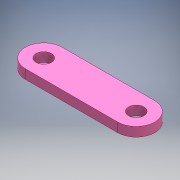
# Autodesk Inventor part: 240614_체인1
Saved by Autodesk Inventor 2016 (Build 200138000, 138)
## iProperties
Created: 2024-06-14
Part Number: 240614_체인1
Material: 일반
Document SubType Name: Modeling
Designer: pc
Density: 1 g/cm^3
Appearance: 분홍색
Author: pc
Autodesk Inventor part; units mm, degrees
ref_plane "YZ Plane" through (0, 0, 0) normal (1, 0, 0) x (0, 1, 0)
ref_plane "XZ Plane" through (0, 0, 0) normal (0, 1, 0) x (-1, 0, 0)
ref_plane "XY Plane" through (0, 0, 0) normal (0, 0, 1) x (1, 0, 0)
sketch "스케치1" plane through (0, 0, 0) normal (0, 0, 1) x (1, 0, 0)
  line L0 (-15, 0) -> (15, 0) construction
  line L1 (-15, -6) -> (15, -6)
  line L2 (15, 6) -> (-15, 6)
  arc A0 (-15, 6) -> (-15, -6) centre (-15, 0) ccw
  arc A1 (15, -6) -> (15, 6) centre (15, 0) ccw
  circle A2 centre (15, 0) radius 2.5
  circle A3 centre (-15, 0) radius 2.5
  point P0 (0, 0)
  dimension "d0" = 12
  dimension "d1" = 30
  dimension "d2" = 5
  dimension "d3" = 5
  constraints: 8 end point, 4 centre point, 4 point on circle, 4 tangent, 2 coincident, 1 horizontal, 1 midpoint, 1 parallel
  measures "d0" distance of L1.end L2.start
  measures "d1" distance of L2.start L2.end
  measures "d2" diameter of A2
  measures "d3" diameter of A3
extrude "돌출1" add sketch "스케치1" along normal blind 3
